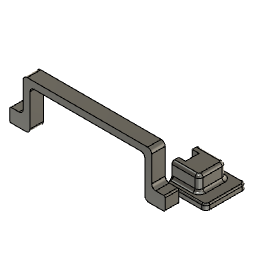
power_supply_support (Autodesk Fusion 360 design; units mm, degrees)
Autodesk Fusion 360 part; units mm, degrees
sketch "Sketch1" plane through (0, 0, 0) normal (0, 1, 0) x (1, 0, 0)
  line L0 (10, 0) -> (10, -30)
  line L1 (10, -30) -> (-75, -30)
  line L2 (-75, -30) -> (-75, 0)
  line L3 (-80, -35) -> (15, -35)
  line L4 (15, -35) -> (15, -10)
  line L5 (-80, -10) -> (-80, -35)
  line L6 (15, 0) -> (10, 0)
  line L7 (-75, 0) -> (-80, 0)
  line L8 (15, -10) -> (25, -10)
  line L9 (25, -10) -> (25, 0)
  line L10 (25, 0) -> (15, 0)
  line L11 (-80, -10) -> (-90, -10)
  line L12 (-90, -10) -> (-90, 0)
  line L13 (-90, 0) -> (-80, 0)
  constraint vertical L0
  constraint horizontal L1
  constraint vertical L2
  constraint horizontal L3
  constraint vertical L4
  constraint horizontal L6
  constraint vertical L5
  constraint collinear L6 L7
  constraint horizontal L8
  constraint vertical L9
  constraint horizontal L10
  constraint horizontal L11
  constraint vertical L12
  constraint horizontal L13
extrude "Extrude1" add sketch "Sketch1" along normal blind 10 makes body 1
fillet "Fillet1" radius 3 1 edges at (15, 5, 35) on bodies 1
fillet "Fillet2" radius 3 1 edges at (-80, 5, 35) on bodies 1
fillet "Fillet3" radius 3 2 edges at (-75, 5, 30) (10, 5, 30) on bodies 1
fillet "Fillet4" radius 3 2 edges at (-75, 5, 0) (10, 5, 0) on bodies 1
fillet "Fillet5" radius 3 2 edges at (-80, 5, 10) (15, 5, 10) on bodies 1
fillet "Fillet6" radius 1 4 edges at (-90, 5, 10) (-90, 5, 0) (25, 5, 0) (25, 5, 10) on bodies 1
sketch "Sketch2" plane through (0, 0, 0) normal (0, 0, 1) x (1, 0, 0)
  line L0 (10, 15) -> (40, 15)
  line L1 (40, 15) -> (40, 45)
  line L2 (40, 45) -> (10, 45)
  line L3 (10, 35) -> (25, 35)
  line L4 (25, 35) -> (25, 25)
  line L5 (25, 25) -> (10, 25)
  line L6 (10, 45) -> (10, 35)
  line L7 (10, 25) -> (10, 15)
  constraint horizontal L0
  constraint vertical L1
  constraint horizontal L2
  constraint vertical L6
  constraint horizontal L3
  constraint vertical L4
  constraint horizontal L5
  constraint collinear L6 L7
extrude "Extrude2" add sketch "Sketch2" along normal blind 4 separate body makes body 2
sketch "Sketch3" plane through (0, 0, 4) normal (0, 0, 1) x (-1, 0, 0)
  line L0 (-10, -25) -> (-10, -15)
  line L1 (-10, -15) -> (-40, -15)
  line L2 (-40, -15) -> (-40, -45)
  line L3 (-40, -45) -> (-10, -45)
  line L4 (-10, -45) -> (-10, -35)
  line L5 (-10, -35) -> (-25, -35)
  line L6 (-25, -35) -> (-25, -25)
  line L7 (-25, -25) -> (-10, -25)
  line L8 (-10, -40) -> (-30, -40)
  line L9 (-30, -40) -> (-30, -20)
  line L10 (-30, -20) -> (-10, -20)
  line L11 (-10, -35) -> (-25, -35)
  line L12 (-25, -35) -> (-25, -25)
  line L13 (-25, -25) -> (-10, -25)
  line L14 (-10, -20) -> (-10, -25)
  line L15 (-10, -35) -> (-10, -40)
  constraint horizontal L8
  constraint vertical L9
  constraint horizontal L10
  constraint vertical L14
  constraint midpoint L4 L8.start
  constraint horizontal L11
  constraint vertical L12
  constraint horizontal L13
  constraint coincident L6.end L7.start
  constraint coincident L4.end L5.start
  constraint collinear L14 L15
extrude "Extrude3" add sketch "Sketch3" along normal blind 6 contours L0 L4 L5 L6 L7 L8 L9 L10 L11 L12 L13 L14 L15 bodies 2
sketch "Sketch4" plane through (0, 0, 10) normal (0, 0, 1) x (-1, 0, 0)
  line L0 (-25, -35) -> (-25, -25)
  line L1 (-25, -25) -> (-10, -25)
  line L2 (-10, -25) -> (-10, -20)
  line L3 (-10, -20) -> (-30, -20)
  line L4 (-30, -20) -> (-30, -40)
  line L5 (-30, -40) -> (-10, -40)
  line L6 (-10, -40) -> (-10, -35)
  line L7 (-10, -35) -> (-25, -35)
  line L8 (-10, -40) -> (-30, -40)
  line L9 (-30, -40) -> (-30, -20)
  line L10 (-30, -20) -> (-10, -20)
  line L11 (-10, -35) -> (-15, -35)
  line L12 (-15, -35) -> (-15, -25)
  line L13 (-15, -25) -> (-10, -25)
  line L14 (-10, -20) -> (-10, -25)
  line L15 (-10, -35) -> (-10, -40)
  constraint horizontal L8
  constraint vertical L9
  constraint horizontal L10
  constraint vertical L14
  constraint coincident L3.end L4.start
  constraint coincident L5.end L6.start
  constraint horizontal L11
  constraint vertical L12
  constraint horizontal L13
  constraint coincident L1 L12.end
  constraint coincident L6.end L7.start
  constraint collinear L14 L15
extrude "Extrude4" add sketch "Sketch4" along normal blind 5 bodies 2
fillet "Fillet7" radius 3 2 edges at (40, 45, 2) (40, 15, 2) on bodies 2
fillet "Fillet8" radius 3 2 edges at (30, 40, 9.5) (30, 20, 9.5) on bodies 2
fillet "Fillet9" radius 1 7 edges at (10, 42.5, 4) (23.5, 15, 4) (39.1213, 15.8787, 4) (40, 30, 4) (39.1213, 44.1213, 4) (23.5, 45, 4) (10, 17.5, 4) on bodies 2
fillet "Fillet10" radius 3 1 edges at (15, 30, 10) on bodies 2
fillet "Fillet11" radius 1 1 edges at (25, 30, 10) on bodies 2
fillet "Fillet12" radius 2 7 edges at (10.2929, 40, 3.7071) (19, 40, 4) (29.1213, 39.1213, 4) (30, 30, 4) (29.1213, 20.8787, 4) (19, 20, 4) (10.2929, 20, 3.7071) on bodies 2
fillet "Fillet13" radius 2 5 edges at (18.5, 20, 15) (29.1213, 20.8787, 15) (30, 30, 15) (29.1213, 39.1213, 15) (18.5, 40, 15) on bodies 2
